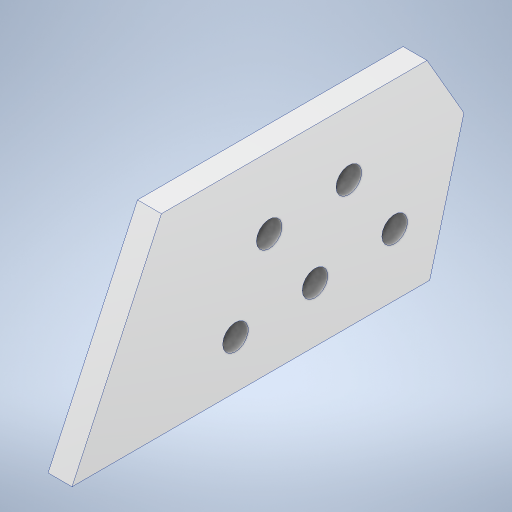
# Autodesk Inventor part: face_gard_right
Saved by Autodesk Inventor 2024.1 (Build 281209000, 209)
## iProperties
Created: 2024-02-25
Part Number: face_gard_right
Material: アルミニウム 6061
Document SubType Name: Sheet Metal
Designer: hibik
Density: 2.7 g/cm^3
Sheet Metal Rule: Default_mm
Appearance: アルミニウム - フラット
Author: hibik
Autodesk Inventor part; units mm, degrees
ref_plane "YZ Plane" through (0, 0, 0) normal (1, 0, 0) x (0, 1, 0)
ref_plane "XZ Plane" through (0, 0, 0) normal (0, 1, 0) x (-1, 0, 0)
ref_plane "XY Plane" through (0, 0, 0) normal (0, 0, 1) x (1, 0, 0)
sketch "スケッチ1" plane through (0, 0, 0) normal (1, 0, 0) x (0, 1, 0)
  line L0 (12, 0) -> (0, 0)
  line L1 (0, 0) -> (0, -25)
  line L2 (0, -25) -> (12, -25)
  line L3 (12, -25) -> (12, 0)
  line L4 (12, 0) -> (0, 5.5957)
  line L5 (0, 5.5957) -> (0, 0)
  line L6 (12, -20) -> (0, -16.7846)
  line L7 (8, -18.9282) -> (12, -16.6188)
  dimension "d11" = 12
  dimension "d12" = 25
  dimension "d14" = 25
  dimension "d15" = 15
  dimension "d16" = 5
  dimension "d17" = 45
  dimension "d18" = 4
  measures "d11" distance of L1.end L2.end
  measures "d12" distance of L2.end L0.start
  measures "d14" angle of L4 L0
  measures "d15" angle of L2 L6
  measures "d16" distance from line of L2 L6.start
  measures "d17" angle of L6 L7
  measures "d18" distance from line of L3 L7.start
extrude "プレート1" add sketch "スケッチ1" along normal blind 1.5 contours L3 L7 L6 L1 L0 | L0 L5 L4
sketch "スケッチ3" plane through (0, 0, 0) normal (-1, 0, 0) x (0, 0, 1)
  circle A0 centre (-6.7433, 7.5315) radius 0.8
  circle A1 centre (-14.5922, 3.8716) radius 0.8
  circle A2 centre (-9.6112, 3.4358) radius 0.8
  circle A3 centre (-4.6303, 3) radius 0.8
  line L0 (-14.5922, 3.8716) -> (-9.6112, 3.4358) construction
  line L1 (-9.6112, 3.4358) -> (-4.6303, 3) construction
  line L2 (-6.7433, 7.5315) -> (-4.6303, 3) construction
  line L3 (0, 12) -> (5.5957, 0) projected
  line L4 (-6.7433, 7.5315) -> (-7.1207, 3.2179) construction
  line L5 (-11.7243, 7.9673) -> (-12.1017, 3.6537) construction
  line L6 (-11.7243, 7.9673) -> (-6.7433, 7.5315) construction
  circle A4 centre (-11.7243, 7.9673) radius 0.8
  line L7 (-6.7433, 7.5315) -> (-4.8683, 8.4059) construction
  line L8 (5.5957, 0) -> (-16.7846, 0) projected
  point P0 (0, 0)
  dimension "d23" = 1.6
  dimension "d26" = 5
  dimension "d29" = 5
  dimension "d30" = 8
  dimension "d31" = 3
  constraints: 14 end point, 5 centre point, 4 equal radius, 3 perpendicular, 2 equal length, 2 midpoint, 1 coincident, 1 collinear, 1 parallel
  measures "d23" diameter of A3
  measures "d26" distance of L0.end L1.end
  measures "d29" distance from line of L1.end L7
  measures "d30" distance between parallel lines of L3 L2
  measures "d31" distance from line of L8 L1.end
extrude "切り取り1" cut sketch "スケッチ3" against normal blind 1.5
equation "\"d29\" = d26"
equation "\"d32\" = Thickness"
equation "\"d0\" = Thickness"
equation "\"BendRadius\" = Thickness"
equation "\"BendReliefWidth\" = Thickness"
equation "\"BendReliefDepth\" = 0.5 * Thickness"
equation "\"CornerReliefSize\" = 4 * Thickness"
equation "\"MinimumRemnant\" = 2 * Thickness"
equation "\"TransitionRadius\" = BendRadius"
equation "\"JacobiRadiusSize\" = BendRadius"
equation "\"GapSize\" = Thickness"
equation "\"Thickness\" = 1.5"
